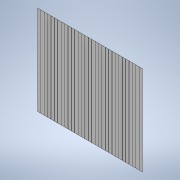
# Autodesk Inventor part: 2.54mmpitchProtoboardDesign_4milheaterwidth
Saved by Autodesk Inventor 2021 (Build 250183000, 183)
## iProperties
Created: 2021-11-09
Part Number: 2.54mmpitchProtoboardDesign_4milheaterwidth
Material: Generic
Document SubType Name: Modeling
Designer: Unit-005
Density: 1 g/cm^3
Appearance: Default
Author: Unit-005
Autodesk Inventor part; units mm, degrees
ref_plane "YZ Plane" through (0, 0, 0) normal (1, 0, 0) x (0, 1, 0)
ref_plane "XZ Plane" through (0, 0, 0) normal (0, 1, 0) x (-1, 0, 0)
ref_plane "XY Plane" through (0, 0, 0) normal (0, 0, 1) x (1, 0, 0)
sketch "Sketch1" plane through (0, 0, 0) normal (0, 0, 1) x (1, 0, 0)
  line L0 (-50.8, 34.8234) -> (50.8, 34.8234)
  line L1 (50.8, 34.8234) -> (50.8, -34.8234)
  line L2 (50.8, -34.8234) -> (-50.8, -34.8234)
  line L3 (-50.8, -34.8234) -> (-50.8, 34.8234)
  line L4 (-50.8, 34.8234) -> (50.8, -34.8234) construction
  line L5 (50.8, 34.8234) -> (-50.8, -34.8234) construction
  point P0 (0, 0)
  dimension "d0" = 101.6
  dimension "d1" = 69.6468
  constraints: 12 end point, 2 midpoint, 2 parallel, 1 horizontal, 1 perpendicular
  measures "d0" distance of L1.end L2.end
  measures "d1" distance of L0.end L1.end
extrude "Extrusion1" add sketch "Sketch1" along normal blind 1.016
sketch "Sketch2" plane through (0, 0, 1.016) normal (0, 0, 1) x (1, 0, 0)
  line L0 (-50.8, -34.8234) -> (50.8, -34.8234) projected
  line L1 (50.8, -34.8234) -> (50.8, 34.8234) projected
  line L2 (50.8, 34.8234) -> (-50.8, 34.8234) projected
  line L3 (-50.8, 34.8234) -> (-50.8, -34.8234) projected
  line L4 (0, -53.34) -> (0, 53.34) projected
  line L5 (-71.12, 0) -> (71.12, 0) projected
  line L6 (-50.8, -34.8234) -> (50.8, -34.8234) projected
  line L7 (-1.27, 34.8234) -> (1.27, 34.8234)
  line L8 (1.27, 34.8234) -> (1.27, -34.8234)
  line L9 (1.27, -34.8234) -> (-1.27, -34.8234)
  line L10 (-1.27, -34.8234) -> (-1.27, 34.8234)
  line L11 (-1.27, 34.8234) -> (1.27, -34.8234) construction
  line L12 (1.27, 34.8234) -> (-1.27, -34.8234) construction
  point P0 (0, 0)
  point P1 (-1.27, 34.8234)
  point P2 (-1.27, -34.8234)
  point P3 (1.27, 34.8234)
  dimension "d4" = 2.54
  constraints: 12 end point, 2 midpoint, 2 parallel, 1 horizontal, 1 perpendicular, 1 point on line
  measures "d4" distance of L8.end L9.end
extrude "Extrusion2" add sketch "Sketch2" along normal blind 0.0381 contours L10 L5 L4 L0 | L4 L5 L8 L0 | L10 L2 L4 L5 | L4 L2 L8 L5
pattern_linear "Rectangular Pattern1" count 31 spacing 2.6416 along (1, 0, 0) of "Extrusion2" first direction both ways yes
sketch "Sketch3" plane through (0, 0, 0) normal (0, 0, -1) x (-1, 0, 0)
  line L0 (71.12, 0) -> (-71.12, 0) projected
  line L1 (0, -53.34) -> (0, 53.34) projected
  line L2 (-50.8, -34.8234) -> (-50.8, 34.8234) projected
  line L3 (50.8, -34.8234) -> (-50.8, -34.8234) projected
  line L4 (50.8, 34.8234) -> (50.8, -34.8234) projected
  line L5 (-50.8, 34.8234) -> (50.8, 34.8234) projected
  line L6 (-50.8, 34.8234) -> (50.8, 34.8234)
  line L7 (50.8, 34.8234) -> (50.8, -34.8234)
  line L8 (50.8, -34.8234) -> (-50.8, -34.8234)
  line L9 (-50.8, -34.8234) -> (-50.8, 34.8234)
  point P0 (0, 0)
  point P1 (-44.8564, 38.1)
  constraints: 8 end point, 2 parallel, 1 horizontal, 1 perpendicular, 1 other
extrude "Extrusion3" cut sketch "Sketch3" against normal up to surface (1.016 mm away)
body "Solid1"
